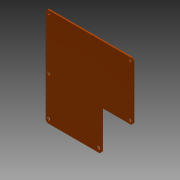
# Autodesk Inventor part: mainboard
Saved by Autodesk Inventor 2015 (Build 190159000, 159)
## iProperties
Created: 2014-10-08
Part Number: mainboard
Material: Phenolic Resin
Document SubType Name: Modeling
Designer: Adam
Density: 1.38 g/cm^3
Appearance: Smooth - Light Orange
Author: Adam
Autodesk Inventor part; units mm, degrees
ref_plane "YZ Plane" through (0, 0, 0) normal (1, 0, 0) x (0, 1, 0)
ref_plane "XZ Plane" through (0, 0, 0) normal (0, 1, 0) x (-1, 0, 0)
ref_plane "XY Plane" through (0, 0, 0) normal (0, 0, 1) x (1, 0, 0)
sketch "Sketch1" plane through (0, 0, 0) normal (0, 0, 1) x (1, 0, 0)
  circle A0 centre (-40.0385, -39) radius 1.75 construction
  line L0 (42.8756, 48.7655) -> (42.8756, -28.7655) construction
  line L1 (42.8756, -28.7655) -> (40.196, -28.7655) construction
  line L2 (40.196, -28.7655) -> (40.196, 48.7655) construction
  line L3 (40.196, 48.7655) -> (42.8756, 48.7655) construction
  spline S0 degree 3 poles (89.6342, -40) (89.6342, -40.307) (89.6036, -40.6423) (89.472, -41.2987) (89.3709, -41.6199) (89.1337, -42.1885) (88.9752, -42.4881) (88.5985, -43.0471) (88.3802, -43.3064) (87.9389, -43.7439) (87.6749, -43.962) (87.1069, -44.3378) (86.8028, -44.4954) (86.2212, -44.7341) (85.8898, -44.8364) (85.2127, -44.9693) (84.8671, -45) (84.5508, -45) knots 0 0 0 0 0.092109 0.092109 0.184218 0.184218 0.276951 0.276951 0.369685 0.369685 0.463374 0.463374 0.557062 0.557062 0.651966 0.651966 0.74687 0.74687 0.74687 0.74687 construction
  line L4 (84.5508, -45) -> (-30, -45) construction
  arc A1 (-33.5564, -43.5146) -> (-30, -45) centre (-30, -40) ccw construction
  spline S1 degree 3 poles (-33.5564, -43.5146) (-33.6039, -43.4665) (-33.657, -43.4242) (-33.7833, -43.3391) (-33.8593, -43.2982) (-34.0668, -43.1998) (-34.2122, -43.1453) (-34.442, -43.0616) (-34.5242, -43.0321) (-34.6067, -43.0012) (-34.6082, -43.0006) (-34.6098, -43) knots -0.12266 -0.12266 -0.12266 -0.12266 -0.100723 -0.100723 -0.073249 -0.073249 -0.02594 -0.02594 0 0 0.000492 0.000492 0.000492 0.000492 construction
  arc A2 (-35.5, -40) -> (-34.6098, -43) centre (-30, -40) ccw construction
  line L5 (-35.5, -40) -> (-35.5, -32) construction
  spline S2 degree 3 poles (-35.5, -32) (-35.3615, -31.8615) (-35.198, -31.6924) (-35.0448, -31.4076) (-35, -31.2614) (-35, -31.134) knots 0 0 0 0 0.058781 0.058781 0.097013 0.097013 0.097013 0.097013 construction
  line L6 (-35, -31.134) -> (-35, -5) construction
  arc A3 (-30, 0) -> (-35, -5) centre (-30, -5) ccw construction
  line L7 (-30, 0) -> (-13.8938, 0) construction
  spline S3 degree 3 poles (-13.8938, 0) (-13.7951, 0) (-13.6962, 0.0043) (-13.4487, 0.0242) (-13.2998, 0.0448) (-12.8834, 0.123) (-12.6198, 0.1971) (-12.1855, 0.3517) (-12.0173, 0.4203) (-11.8433, 0.4975) (-11.8405, 0.4988) (-11.8377, 0.5) knots -0.215254 -0.215254 -0.215254 -0.215254 -0.185183 -0.185183 -0.139614 -0.139614 -0.056186 -0.056186 0 0 0.000914 0.000914 0.000914 0.000914 construction
  line L8 (-11.8377, 0.5) -> (-3, 0.5) construction
  arc A4 (-3, 0.5) -> (-0.5, 3) centre (-3, 3) ccw construction
  line L9 (-0.5, 3) -> (-0.5, 63) construction
  arc A5 (1.8377, 67.5) -> (-0.5, 63) centre (5, 63) ccw construction
  spline S4 degree 3 poles (1.8377, 67.5) (1.8408, 67.5006) (1.8439, 67.5012) (2.091, 67.5495) (2.4162, 67.6049) (2.8871, 67.6848) (3.1573, 67.7302) (3.5823, 67.8102) (3.7456, 67.8428) (3.9031, 67.8782) knots -0.188965 -0.188965 -0.188965 -0.188965 -0.188229 -0.188229 -0.130201 -0.130201 -0.048433 -0.048433 0 0 0 0 construction
  arc A6 (5, 68) -> (3.9031, 67.8782) centre (5, 63) ccw construction
  line L10 (5, 68) -> (84.5508, 68) construction
  spline S5 degree 3 poles (84.5508, 68) (84.8671, 68) (85.2127, 67.9693) (85.8898, 67.8364) (86.2212, 67.7341) (86.8028, 67.4954) (87.1069, 67.3378) (87.6749, 66.962) (87.9389, 66.7439) (88.3802, 66.3064) (88.5985, 66.0471) (88.9752, 65.4881) (89.1337, 65.1885) (89.3709, 64.6199) (89.472, 64.2987) (89.6036, 63.6423) (89.6342, 63.307) (89.6342, 63) knots -0.74687 -0.74687 -0.74687 -0.74687 -0.651966 -0.651966 -0.557062 -0.557062 -0.463374 -0.463374 -0.369685 -0.369685 -0.276951 -0.276951 -0.184218 -0.184218 -0.092109 -0.092109 0 0 0 0 construction
  line L11 (89.6342, 63) -> (89.6342, -40) construction
  line L12 (-34.6098, -43) -> (-43, -43) construction
  arc A7 (-44.5, -41.5) -> (-43, -43) centre (-43, -41.5) ccw construction
  line L13 (-44.5, -41.5) -> (-44.5, -33.5) construction
  arc A8 (-43, -32) -> (-44.5, -33.5) centre (-43, -33.5) ccw construction
  line L14 (-43, -32) -> (-35.5, -32) construction
  arc A9 (-11.8377, 0.5) -> (-9.5, 5) centre (-15, 5) ccw construction
  line L15 (-9.5, 5) -> (-9.5, 8.6603) construction
  arc A10 (-8.8971, 10.9103) -> (-9.5, 8.6603) centre (-5, 8.6603) ccw construction
  line L16 (-8.8971, 10.9103) -> (-2.2369, 22.4462) construction
  arc A11 (-2.2369, 22.4462) -> (-1.5, 25.1962) centre (-7, 25.1962) ccw construction
  line L17 (-1.5, 25.1962) -> (-1.5, 42.8038) construction
  arc A12 (-1.5, 42.8038) -> (-2.2369, 45.5538) centre (-7, 42.8038) ccw construction
  line L18 (-2.2369, 45.5538) -> (-8.8971, 57.0897) construction
  arc A13 (-9.5, 59.3397) -> (-8.8971, 57.0897) centre (-5, 59.3397) ccw construction
  line L19 (-9.5, 59.3397) -> (-9.5, 65) construction
  arc A14 (-7, 67.5) -> (-9.5, 65) centre (-7, 65) ccw construction
  line L20 (1.8377, 67.5) -> (-7, 67.5) construction
  arc A15 (4.1416, 64.7033) -> (3.0926, 63) centre (5, 63) ccw construction
  line L21 (3.0926, 63) -> (3.0926, 3) construction
  spline S6 degree 3 poles (3.0926, 3) (3.0926, 2.7157) (3.051, 2.4082) (2.8879, 1.813) (2.7678, 1.5249) (2.4803, 0.9673) (2.276, 0.6516) (1.8113, 0.0638) (1.5508, -0.2083) (1.0345, -0.6709) (0.7291, -0.9038) (0.0797, -1.307) (-0.2644, -1.477) (-0.9, -1.7256) (-1.2494, -1.8303) (-1.962, -1.9676) (-2.3251, -2) (-2.6576, -2) knots 1.5371 1.5371 1.5371 1.5371 1.622376 1.622376 1.707652 1.707652 1.810613 1.810613 1.913573 1.913573 2.018567 2.018567 2.12356 2.12356 2.223299 2.223299 2.323037 2.323037 2.323037 2.323037 construction
  line L22 (-2.6576, -2) -> (-30, -2) construction
  arc A16 (-30, -2) -> (-33, -5) centre (-30, -5) ccw construction
  line L23 (-33, -5) -> (-33, -40) construction
  arc A17 (-33, -40) -> (-30, -43) centre (-30, -40) ccw construction
  line L24 (-30, -43) -> (84.5508, -43) construction
  spline S7 degree 3 poles (84.5508, -43) (84.9307, -43) (85.3782, -42.9124) (86.0771, -42.6259) (86.4531, -42.3779) (86.9836, -41.8526) (87.233, -41.4836) (87.5181, -40.8014) (87.6053, -40.3682) (87.6053, -40) knots -0.448416 -0.448416 -0.448416 -0.448416 -0.334429 -0.334429 -0.221821 -0.221821 -0.110466 -0.110466 0 0 0 0 construction
  line L25 (87.6053, -40) -> (87.6053, -27.0969) construction
  line L26 (87.6053, -27.0969) -> (86.08, -27.0969) construction
  line L27 (86.08, -27.0969) -> (86.08, -25.2969) construction
  line L28 (86.08, -25.2969) -> (87.6053, -25.2969) construction
  line L29 (87.6053, -25.2969) -> (87.6053, -23.4969) construction
  line L30 (87.6053, -23.4969) -> (86.08, -23.4969) construction
  line L31 (86.08, -23.4969) -> (86.08, -21.6969) construction
  line L32 (86.08, -21.6969) -> (87.6053, -21.6969) construction
  line L33 (87.6053, -21.6969) -> (87.6053, 36.1031) construction
  line L34 (87.6053, 36.1031) -> (86.08, 36.1031) construction
  line L35 (86.08, 36.1031) -> (86.08, 37.9031) construction
  line L36 (86.08, 37.9031) -> (87.6053, 37.9031) construction
  line L37 (87.6053, 37.9031) -> (87.6053, 39.7031) construction
  line L38 (87.6053, 39.7031) -> (86.08, 39.7031) construction
  line L39 (86.08, 39.7031) -> (86.08, 41.5031) construction
  line L40 (86.08, 41.5031) -> (87.6053, 41.5031) construction
  line L41 (87.6053, 41.5031) -> (87.6053, 63) construction
  spline S8 degree 3 poles (87.6053, 63) (87.6053, 63.3682) (87.5181, 63.8014) (87.233, 64.4836) (86.9836, 64.8526) (86.4531, 65.3779) (86.0771, 65.6259) (85.3782, 65.9124) (84.9307, 66) (84.5508, 66) knots 0 0 0 0 0.110466 0.110466 0.221821 0.221821 0.334429 0.334429 0.448416 0.448416 0.448416 0.448416 construction
  line L42 (84.5508, 66) -> (9.0869, 66) construction
  spline S9 degree 3 poles (9.0869, 66) (8.2981, 66) (7.4479, 65.8733) (5.7921, 65.4298) (4.9854, 65.1168) (4.2322, 64.7487) (4.1871, 64.7263) (4.1416, 64.7033) knots 0.547089 0.547089 0.547089 0.547089 0.783714 0.783714 1.02034 1.02034 1.035217 1.035217 1.035217 1.035217 construction
  circle A18 centre (-5, 63) radius 1.25 construction
  circle A19 centre (-5, 5) radius 1.25 construction
  circle A20 centre (-95.5, 63) radius 1.4224 construction
  circle A21 centre (-95.5, 5) radius 1.4224 construction
  line L43 (93.4273, 72) -> (93.4273, 74.5) construction
  line L44 (93.4273, 74.5) -> (92.1643, 74.5) construction
  line L45 (92.1643, 74.5) -> (92.1643, 76.5) construction
  line L46 (92.1643, 76.5) -> (94.6893, 76.5) construction
  line L47 (94.6893, 76.5) -> (94.6893, -53.5) construction
  line L48 (94.6893, -53.5) -> (92.1643, -53.5) construction
  line L49 (92.1643, -53.5) -> (92.1643, -51.5) construction
  line L50 (92.1643, -51.5) -> (93.4273, -51.5) construction
  line L51 (93.4273, -51.5) -> (93.4273, -49) construction
  line L52 (93.4273, -49) -> (90.6469, -49) construction
  line L53 (90.6469, -49) -> (90.6469, -47) construction
  line L54 (90.6469, -47) -> (92.1643, -47) construction
  line L55 (92.1643, -47) -> (92.1643, 70) construction
  line L56 (92.1643, 70) -> (90.6469, 70) construction
  line L57 (90.6469, 70) -> (90.6469, 72) construction
  line L58 (90.6469, 72) -> (93.4273, 72) construction
  line L59 (-103.5043, 74.5) -> (-103.5043, 72) construction
  line L60 (-103.5043, 72) -> (-100.7239, 72) construction
  line L61 (-100.7239, 72) -> (-100.7239, 70) construction
  line L62 (-100.7239, 70) -> (-102.2413, 70) construction
  line L63 (-102.2413, 70) -> (-102.2413, 63.75) construction
  line L64 (-102.2413, 63.75) -> (-98.6339, 63.75) construction
  arc A22 (-98.6339, 62.25) -> (-98.6339, 63.75) centre (-95.5, 63) ccw construction
  line L65 (-98.6339, 62.25) -> (-102.2413, 62.25) construction
  line L66 (-102.2413, 62.25) -> (-102.2413, 5.75) construction
  line L67 (-102.2413, 5.75) -> (-98.6339, 5.75) construction
  arc A23 (-98.6339, 4.25) -> (-98.6339, 5.75) centre (-95.5, 5) ccw construction
  line L68 (-98.6339, 4.25) -> (-102.2413, 4.25) construction
  line L69 (-102.2413, 4.25) -> (-102.2413, -47) construction
  line L70 (-102.2413, -47) -> (-100.7239, -47) construction
  line L71 (-100.7239, -47) -> (-100.7239, -49) construction
  line L72 (-100.7239, -49) -> (-103.5043, -49) construction
  line L73 (-103.5043, -49) -> (-103.5043, -51.5) construction
  line L74 (-103.5043, -51.5) -> (-102.2413, -51.5) construction
  line L75 (-102.2413, -51.5) -> (-102.2413, -53.5) construction
  line L76 (-102.2413, -53.5) -> (-104.7663, -53.5) construction
  line L77 (-104.7663, -53.5) -> (-104.7663, 76.5) construction
  line L78 (-104.7663, 76.5) -> (-102.2413, 76.5) construction
  line L79 (-102.2413, 76.5) -> (-102.2413, 74.5) construction
  line L80 (-102.2413, 74.5) -> (-103.5043, 74.5) construction
  line L81 (-102.2413, 63.75) -> (-102.2413, 62.25) construction
  line L82 (-102.2413, 5.75) -> (-102.2413, 4.25) construction
  line L83 (-98.7224, 66.2224) -> (-1.5, 66.2224)
  line L84 (-1.5, 66.2224) -> (-1.5, 1.5)
  line L85 (-1.5, 1.5) -> (-36.5385, 1.5)
  line L86 (-98.7224, 1.5) -> (-98.7224, 66.2224)
  line L87 (-36.5385, 1.5) -> (-36.5385, -43.5)
  line L88 (-36.5385, -43.5) -> (-98.7224, -43.5)
  line L89 (-98.7224, -43.5) -> (-98.7224, 1.5)
  circle A24 centre (-95.5, 5) radius 1.75
  circle A25 centre (-95.5, 63) radius 1.75
  circle A26 centre (-5, 63) radius 1.75
  circle A27 centre (-5, 5) radius 1.75
  circle A28 centre (-40.0385, -39) radius 1.75
  circle A29 centre (-95.5, -39) radius 1.4224 construction
  circle A30 centre (-95.5, -39) radius 1.75
  point P0 (0, 0)
  dimension "d0" = 3.5
  dimension "d1" = 3.5
  dimension "d2" = 3.5
  dimension "d3" = 4.5
  dimension "d5" = 3.5
  constraints: 180 end point, 41 horizontal, 41 vertical, 38 point on circle, 30 centre point, 6 coincident, 5 equal radius, 4 parallel, 2 tangent, 1 collinear, 1 perpendicular, 180 other
  measures "d0" distance from line of A18.centre L84
  measures "d1" distance from line of L85 A19.centre
  measures "d2" distance from line of L87 A0.centre
  measures "d3" distance from line of L88 A0.centre
  measures "d5" diameter of A25
extrude "Extrusion1" add sketch "Sketch1" along normal blind 1.5
chamfer "Chamfer1" distance 2 angle 45 6 edges at (-98.7224, -43.5, 0.75) (-36.5385, -43.5, 0.75) (-36.5385, 1.5, 0.75) (-1.5, 1.5, 0.75) (-1.5, 66.2224, 0.75) (-98.7224, 66.2224, 0.75)
body "Solid1"
